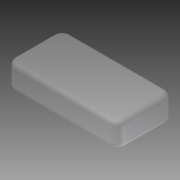
# Autodesk Inventor part: esc
Saved by Autodesk Inventor 2012 (Build 160160000, 160)
## iProperties
Created: 2014-07-18
Part Number: esc
Material: Default
Document SubType Name: Modeling
Designer: Anon
Density: 1 g/cm^3
Author: Anon
Autodesk Inventor part; units mm, degrees
ref_plane "YZ Plane" through (0, 0, 0) normal (1, 0, 0) x (0, 1, 0)
ref_plane "XZ Plane" through (0, 0, 0) normal (0, 1, 0) x (-1, 0, 0)
ref_plane "XY Plane" through (0, 0, 0) normal (0, 0, 1) x (1, 0, 0)
sketch "Sketch1" plane through (0, 0, 0) normal (0, 0, 1) x (1, 0, 0)
  line L0 (-25, 12.5) -> (25, 12.5)
  line L1 (25, 12.5) -> (25, -12.5)
  line L2 (25, -12.5) -> (-25, -12.5)
  line L3 (-25, -12.5) -> (-25, 12.5)
  point P0 (0, 0)
  dimension "d0" = 50
  dimension "d1" = 25
  dimension "d2" = 25
  dimension "d3" = 12.5
  constraints: 8 end point, 2 parallel, 1 horizontal, 1 perpendicular
  measures "d0" distance of L1.end L2.end
  measures "d1" distance of L0.end L1.end
  measures "d2" distance from line of point (0, 0) L3
  measures "d3" distance from line of point (0, 0) L0
extrude "Extrusion1" add sketch "Sketch1" along normal blind 11
fillet "Fillet1" radius 2 4 edges at (25, -12.5, 5.5) (25, 12.5, 5.5) (-25, 12.5, 5.5) (-25, -12.5, 5.5)
fillet "Fillet2" radius 2 16 edges at (-25, 0, 11) (-24.4142, 11.9142, 11) (0, 12.5, 11) (24.4142, 11.9142, 11) (25, 0, 11) (24.4142, -11.9142, 11) (0, -12.5, 11) (-24.4142, -11.9142, 11) (-24.4142, -11.9142, 0) (-25, 0, 0) (-24.4142, 11.9142, 0) (0, 12.5, 0) (24.4142, 11.9142, 0) (25, 0, 0) (24.4142, -11.9142, 0) (0, -12.5, 0)
body "Solid1"
